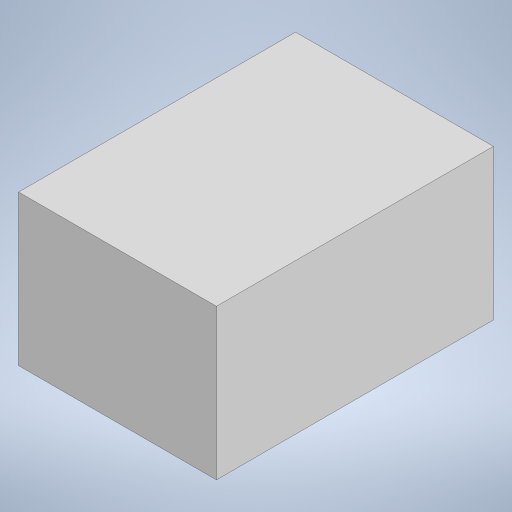
# Autodesk Inventor part: but
Saved by Autodesk Inventor 2023.4 (Build 274418000, 418)
## iProperties
Created: 2024-08-02
Part Number: but
Material: Generic
Document SubType Name: Modeling
Designer: komputer
Density: 1 g/cm^3
Appearance: Default
Author: komputer
Autodesk Inventor part; units mm, degrees
ref_plane "YZ Plane" through (0, 0, 0) normal (1, 0, 0) x (0, 1, 0)
ref_plane "XZ Plane" through (0, 0, 0) normal (0, 1, 0) x (-1, 0, 0)
ref_plane "XY Plane" through (0, 0, 0) normal (0, 0, 1) x (1, 0, 0)
sketch "Sketch1" plane through (0, 0, 0) normal (1, 0, 0) x (0, 1, 0)
  line L0 (4.5638, 12.6931) -> (-3.0362, 12.6931)
  line L1 (-3.0362, 12.6931) -> (-3.0362, -1.3069)
  line L2 (-3.0362, -1.3069) -> (4.5638, -1.3069)
  line L3 (4.5638, -1.3069) -> (4.5638, 12.6931)
  point P0 (0, 0)
  dimension "d0" = 7.6
  dimension "d1" = 14
  constraints: 8 end point, 2 parallel, 1 horizontal, 1 perpendicular
  measures "d0" distance of L2.end L1.end
  measures "d1" distance of L1.end L0.end
extrude "Extrusion1" add sketch "Sketch1" along normal blind 7
sketch "Sketch2" plane through (0, 0, 0) normal (-1, 0, 0) x (0, 0, 1)
  line L0 (12.6931, -3.0362) -> (-1.3069, -3.0362) projected
  line L1 (12.6931, 4.5638) -> (12.6931, -3.0362) projected
  line L2 (-1.3069, 4.5638) -> (12.6931, 4.5638) projected
  line L3 (-1.3069, -3.0362) -> (-1.3069, 4.5638) projected
  point P0 (0, 0)
extrude "Extrusion2" add sketch "Sketch2" along normal blind 3
body "Solid1"
